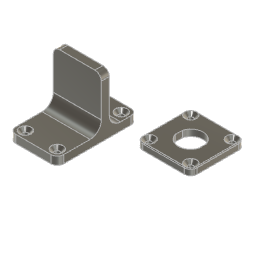
COCKPIT HANDHELD LIGHT BRACKET v3 (Autodesk Fusion 360 design; units mm, degrees)
Autodesk Fusion 360 part; units mm, degrees
sketch "Sketch1" plane through (0, 0, 0) normal (1, 0, 0) x (0, 1, 0)
  line L0 (2.5, -16) -> (-2.5, -16)
  line L1 (-2.5, -16) -> (-2.5, 16)
  line L2 (-2.5, 16) -> (2.5, 16)
  line L3 (2.5, 16) -> (2.5, -16)
  line L4 (2.5, -16) -> (-2.5, 16) construction
  line L5 (-2.5, -16) -> (2.5, 16) construction
  line L6 (0, -16) -> (0, -21)
  line L7 (0, -16) -> (-30, -16)
  line L8 (-30, -16) -> (-30, -21)
  line L9 (-30, -21) -> (0, -21)
  line L10 (0, -21) -> (0, -16)
  line L11 (0, -16) -> (20, -16)
  line L12 (20, -16) -> (20, -21)
  line L13 (20, -21) -> (0, -21)
  line L14 (0, -21) -> (0, -16)
  dimension "d1" = 5
  dimension "d2" = 32
  dimension "d3" = 5
  dimension "d4" = 30
  dimension "d5" = 5
  dimension "d6" = 20
  dimension "d7" = 5
  constraint horizontal L0
  constraint perpendicular L0 L1
  constraint parallel L0 L2
  constraint parallel L1 L3
  constraint coincident L4 origin
  constraint coincident L5 origin
  constraint midpoint L0 L6.start
  constraint perpendicular L0 L6
  constraint horizontal L7
  constraint vertical L8
  constraint horizontal L9
  constraint vertical L10
  constraint horizontal L11
  constraint vertical L12
  constraint horizontal L13
  constraint vertical L14
  measures "d1" distance of L1.end L2.end
  measures "d2" distance of L0.end L1.end
  measures "d3" distance of L6.start L6.end
  measures "d4" distance of L6.start L7.end
  measures "d5" distance of L6.start L6.end
  measures "d6" distance of L6.start L11.end
  measures "d7" distance of L6.start L6.end
extrude "Extrude1" add sketch "Sketch1" against normal blind 30 makes body 1
sketch "Sketch2" plane through (0, 0, -21) normal (0, 0, -1) x (1, 0, 0)
  line L0 (0, -20) -> (0, 30)
  line L1 (0, 30) -> (-30, 30)
  line L2 (-30, 30) -> (-30, -20)
  line L3 (-30, -20) -> (0, -20)
  line L4 (-5, -15) -> (-25, 25) construction
  line L5 (-25, -15) -> (-5, 25) construction
  circle A0 centre (-25, 25) radius 1.65
  circle A1 centre (-5, 25) radius 1.65
  circle A2 centre (-5, -15) radius 1.65
  circle A3 centre (-25, -15) radius 1.65
  point P0 (-15, 5)
  dimension "d10" = 20
  dimension "d11" = 40
  dimension "d12" = 3.3
  dimension "d13" = 3.3
  dimension "d14" = 3.3
  dimension "d15" = 3.3
  constraint coincident L4 P0
  constraint coincident L5 P0
  constraint coincident L4.end A0.centre
  constraint coincident L5.end A1.centre
  constraint coincident L4.start A2.centre
  constraint coincident L5.start A3.centre
  measures "d10" distance of L4.end L5.end
  measures "d11" distance of L5.start L4.end
  measures "d12" diameter of A0
  measures "d13" diameter of A1
  measures "d14" diameter of A2
  measures "d15" diameter of A3
extrude "Extrude2" cut sketch "Sketch2" against normal blind 5 contours A0 | A1 | A2 | A3 bodies 1
chamfer "Chamfer1" distance 2 angle 45 4 edges at (-26.5383, -24.4033, -16) (-6.5383, -24.4033, -16) (-6.5383, 15.5967, -16) (-26.5383, 15.5967, -16) on bodies 1
fillet "Fillet1" radius 4 4 edges at (-30, -30, -18.5) (0, -30, -18.5) (0, 20, -18.5) (-30, 20, -18.5) on bodies 1
fillet "Fillet2" radius 4 2 edges at (-30, 0, 16) (0, 0, 16) on bodies 1
fillet "Fillet3" radius 7 2 edges at (-15, -2.5, -16) (-15, 2.5, -16) on bodies 1
sketch "Sketch3" plane through (0, 0, 0) normal (0, 0, 1) x (1, 0, 0)
  circle A0 centre (51.3856, 2.0286) radius 7.75
  line L0 (68.3856, -14.9714) -> (34.3856, -14.9714)
  line L1 (34.3856, -14.9714) -> (34.3856, 19.0286)
  line L2 (34.3856, 19.0286) -> (68.3856, 19.0286)
  line L3 (68.3856, 19.0286) -> (68.3856, -14.9714)
  line L4 (68.3856, -14.9714) -> (34.3856, 19.0286) construction
  line L5 (34.3856, -14.9714) -> (68.3856, 19.0286) construction
  line L6 (64.3856, -10.9714) -> (38.3856, -10.9714)
  line L7 (38.3856, -10.9714) -> (38.3856, 15.0286)
  line L8 (38.3856, 15.0286) -> (64.3856, 15.0286)
  line L9 (64.3856, 15.0286) -> (64.3856, -10.9714)
  line L10 (64.3856, -10.9714) -> (38.3856, 15.0286) construction
  line L11 (38.3856, -10.9714) -> (64.3856, 15.0286) construction
  line L12 (58.7856, -7.9714) -> (43.9856, -7.9714)
  line L13 (43.9856, -7.9714) -> (43.9856, 12.0286)
  line L14 (43.9856, 12.0286) -> (58.7856, 12.0286)
  line L15 (58.7856, 12.0286) -> (58.7856, -7.9714)
  line L16 (58.7856, -7.9714) -> (43.9856, 12.0286) construction
  line L17 (43.9856, -7.9714) -> (58.7856, 12.0286) construction
  circle A1 centre (38.3856, 15.0286) radius 1.65
  circle A2 centre (64.3856, 15.0286) radius 1.65
  circle A3 centre (64.3856, -10.9714) radius 1.65
  circle A4 centre (38.3856, -10.9714) radius 1.65
  point P0 (51.3856, 2.0286)
  point P1 (51.3856, 2.0286)
  point P2 (51.3856, 2.0286)
  dimension "d55" = 15.5
  dimension "d56" = 34
  dimension "d57" = 34
  dimension "d58" = 26
  dimension "d59" = 26
  dimension "d60" = 14.8
  dimension "d61" = 20
  dimension "d62" = 3.3
  dimension "d63" = 3.3
  dimension "d64" = 3.3
  dimension "d65" = 3.3
  constraint horizontal L0
  constraint perpendicular L0 L1
  constraint parallel L0 L2
  constraint parallel L1 L3
  constraint coincident L4 P2
  constraint coincident L5 P2
  constraint coincident P2 P0
  constraint horizontal L6
  constraint perpendicular L6 L7
  constraint parallel L6 L8
  constraint parallel L7 L9
  constraint coincident L10 P2
  constraint coincident L11 P2
  constraint horizontal L12
  constraint perpendicular L12 L13
  constraint parallel L12 L14
  constraint parallel L13 L15
  constraint coincident L16 P2
  constraint coincident L17 P2
  constraint coincident P2 P1
  constraint coincident L7.end L8.start
  constraint coincident L8.end L9.start
  constraint coincident L6.start L9.end
  constraint coincident L6.end L7.start
  measures "d55" diameter of A0
  measures "d56" distance of L1.end L2.end
  measures "d57" distance of L0.end L1.end
  measures "d58" distance of L7.end L8.end
  measures "d59" distance of L6.end L7.end
  measures "d60" distance of L13.end L14.end
  measures "d61" distance of L12.end L13.end
  measures "d62" diameter of A1
  measures "d63" diameter of A2
  measures "d64" diameter of A3
  measures "d65" diameter of A4
extrude "Extrude8" add sketch "Sketch3" along normal blind 4 separate body contours A0 L15 | A0 L13 L14 L15 | A0 L12 L13 L15 | A0 L13 | L0 L1 L2 L3 | L6 L7 L8 L9 A1 A2 A3 A4 makes body 2
chamfer "Chamfer4" distance 2 angle 45 4 edges at (36.8473, 15.6252, 4) (36.8473, -10.3748, 4) (62.8473, -10.3748, 4) (62.8473, 15.6252, 4) on bodies 2
fillet "Fillet7" radius 4 4 edges at (34.3856, -14.9714, 2) (68.3856, -14.9714, 2) (34.3856, 19.0286, 2) (68.3856, 19.0286, 2) on bodies 2
fillet "Fillet8" radius 0.5 8 edges at (67.214, 17.857, 4) (51.3856, 19.0286, 4) (35.5572, 17.857, 4) (34.3856, 2.0286, 4) (35.5572, -13.7999, 4) (51.3856, -14.9714, 4) (67.214, -13.7999, 4) (68.3856, 2.0286, 4) on bodies 2
named bodies: "HOLDER", "CONNECTOR MOUNT"
